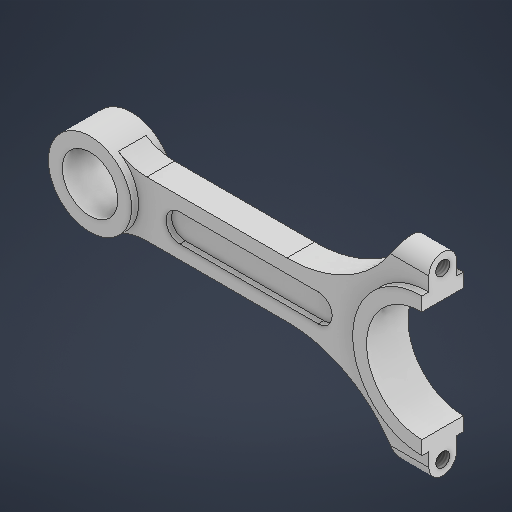
# Autodesk Inventor part: connectingrod
Saved by Autodesk Inventor 2026.1 (Build 301233020, 233B)
## iProperties
Created: 2025-09-17
Part Number: connectingrod
Material: Generic
Document SubType Name: Modeling
Designer: ender
Density: 1 g/cm^3
Appearance: Default
Author: ender
Autodesk Inventor part; units mm, degrees
ref_plane "YZ Plane" through (0, 0, 0) normal (1, 0, 0) x (0, 1, 0)
ref_plane "XZ Plane" through (0, 0, 0) normal (0, 1, 0) x (-1, 0, 0)
ref_plane "XY Plane" through (0, 0, 0) normal (0, 0, 1) x (1, 0, 0)
sketch "Sketch1" plane through (0, 0, 0) normal (0, 0, 1) x (1, 0, 0)
  circle A0 centre (0, 0) radius 19.05
  arc A1 (152.4, 25.4) -> (152.4, -25.4) centre (152.4, 0) ccw
  line L0 (22.8953, 12.7) -> (87.2347, 12.7)
  line L1 (87.2347, -12.7) -> (22.8953, -12.7)
  line L2 (138.43, 44.45) -> (152.4, 44.45)
  line L3 (152.4, -44.45) -> (138.43, -44.45)
  arc A2 (138.43, -44.45) -> (87.2347, -12.7) centre (87.2347, -69.85) ccw
  arc A3 (87.2347, 12.7) -> (138.43, 44.45) centre (87.2347, 69.85) ccw
  arc A4 (9.8123, 16.3286) -> (22.8953, 12.7) centre (22.8953, 38.1) ccw
  arc A5 (22.8953, -12.7) -> (9.8123, -16.3286) centre (22.8953, -38.1) ccw
  line L4 (152.4, 44.45) -> (152.4, 25.4)
  line L5 (152.4, -25.4) -> (152.4, -44.45)
  circle A6 centre (0, 0) radius 12.7
  arc A7 (152.4, 31.75) -> (152.4, -31.75) centre (152.4, 0) ccw
  dimension "d0" = 38.1
  dimension "d2" = 152.4
  dimension "d3" = 25.4
  dimension "d4" = 25.4
  dimension "d5" = 57.15
  dimension "d6" = 13.97
  dimension "d7" = 88.9
  dimension "d8" = 25.4
  dimension "d9" = 31.75
  dimension "d10" = 25.4
  constraints: 14 point on circle, 12 end point, 8 centre point, 6 tangent, 3 coincident, 3 equal length, 3 point on line, 2 equal radius, 2 horizontal, 2 parallel, 2 perpendicular, 1 collinear, 1 horizontal alignment
  measures "d0" diameter of A0
  measures "d2" distance of A0.centre A1.centre
  measures "d3" distance between parallel lines of L0 L1
  measures "d4" radius of A5
  measures "d5" radius of A3
  measures "d6" distance of L2.start L2.end
  measures "d7" distance of L3.start L2.end
  measures "d8" radius of A1
  measures "d9" radius of A7
  measures "d10" diameter of A6
extrude "Extrusion1" add sketch "Sketch1" along normal mid plane 12.7 contours A0 A4 L0 A3 L2 L4 A7 L5 L3 A2 L1 A5
extrude "Extrusion2" add sketch "Sketch1" along normal mid plane 19.05 contours A0 | L4 A1 L5 A7
sketch "Sketch2" plane through (0, 0, 6.35) normal (0, 0, 1) x (1, 0, 0)
  circle A0 centre (38.1, 0) radius 6.35
  circle A1 centre (101.6, 0) radius 6.35
  line L0 (38.1, 6.35) -> (101.6, 6.35)
  line L1 (38.1, -6.35) -> (101.6, -6.35)
  point P0 (0, 0)
  dimension "d15" = 38.1
  dimension "d16" = 63.5
  dimension "d17" = 12.7
  constraints: 4 end point, 4 point on circle, 2 centre point, 2 horizontal alignment, 2 tangent, 1 equal radius
  measures "d15" distance of point (0, 0) A0.centre
  measures "d16" distance of A1.centre A0.centre
  measures "d17" distance between parallel lines of L1 L0
extrude "Extrusion3" cut sketch "Sketch2" against normal blind 2.54
mirror "Mirror1" about plane through (0, 0, 0) normal (0, 0, 1) of "Extrusion3"
fillet "Fillet1" radius 6.35 4 edges at (145.415, 44.45, 6.35) (145.415, 44.45, -6.35) (145.415, -44.45, 6.35) (145.415, -44.45, -6.35)
sketch "Sketch3" plane through (152.4, -31.75, -9.525) normal (1, 0, 0) x (0, 0, -1)
  arc A0 (-3.175, 69.85) -> (-15.875, 69.85) centre (-9.525, 69.85) ccw projected
  arc A1 (-15.875, -6.35) -> (-3.175, -6.35) centre (-9.525, -6.35) ccw projected
  line L0 (-3.175, 0) -> (-3.175, -6.35) projected
  line L1 (-15.875, -6.35) -> (-15.875, 0) projected
  line L2 (-19.05, 0) -> (-19.05, 6.35) projected
  line L3 (0, 6.35) -> (-19.05, 6.35) projected
  line L4 (0, 6.35) -> (0, 0) projected
  arc A2 (-15.875, -6.35) -> (-3.175, -6.35) centre (-9.525, -6.35) ccw projected
  line L5 (-3.175, 0) -> (-3.175, -6.35) projected
  line L6 (0, 0) -> (-3.175, 0) projected
  line L7 (0, 6.35) -> (0, 0) projected
  line L8 (0, 6.35) -> (-19.05, 6.35) projected
  line L9 (-19.05, 0) -> (-19.05, 6.35) projected
  line L10 (-15.875, 0) -> (-19.05, 0) projected
  line L11 (-15.875, -6.35) -> (-15.875, 0) projected
  point P0 (-9.525, 31.75)
hole "Hole1" at (152.4, 38.1, 0) at (152.4, -38.1, 0) direction (-1, 0, 0) diameter 6.35 end through all
thread "Thread1" size "1/4-20 UNC" class "2B" standard "ANSI Unified Screw Threads" full length
thread "Thread2" size "1/4-20 UNC" class "2B" standard "ANSI Unified Screw Threads" full length
body "Solid1"
